Mast 3 (Autodesk Fusion 360 design; units mm, degrees)
Autodesk Fusion 360 part; units mm, degrees
sketch "Sketch1" plane through (0, 0, 0) normal (0, 0, 1) x (1, 0, 0)
  circle A0 centre (0, 0) radius 33
  circle A1 centre (0, 0) radius 32
  circle A2 centre (0, 0) radius 30
  circle A3 centre (0, 0) radius 16.2
  dimension "d1" = 66
  dimension "d2" = -1
  dimension "d3" = -3
  dimension "d10" = 60
  dimension "d15" = 32.4
  constraint coincident A0.centre A1.centre
  measures "d1" diameter of A0
  measures "d10" diameter of A2
  measures "d15" diameter of A3
extrude "Extrude1" add sketch "Sketch1" along normal blind 17 contours A0 | A1 | A2
extrude "Extrude2" cut sketch "Sketch1" along normal blind 15 contours A2 | A3
extrude "Extrude3" cut sketch "Sketch1" along normal blind 2 contours A1
sketch "Sketch2" plane through (0, 0, 15) normal (0, 0, -1) x (1, 0, 0)
  circle A0 centre (0, 0) radius 30
  line L0 (0, 0) -> (-30, 0) construction
  line L1 (-30, 5) -> (-29.5804, 5)
  line L2 (-16, 2.6667) -> (-16, -2.6667)
  line L3 (-29.5804, -5) -> (-30, -5)
  line L4 (-30, -5) -> (-30, 5)
  circle A1 centre (0, 0) radius 16.2
  line L5 (-30, 5) -> (0, 0) construction
  line L6 (-30, -5) -> (0, 0) construction
  line L7 (-30, 5) -> (-16, 2.6667)
  line L8 (-30, -5) -> (-16, -2.6667)
  dimension "d11" = 10
  dimension "d16" = 14
  constraint coincident A0.centre L0.start
  constraint coincident A0 L0.end
  constraint horizontal L0
  constraint horizontal L1
  constraint vertical L2
  constraint horizontal L3
  constraint vertical L4
  constraint coincident L0.end L4
  constraint midpoint L0.end L4
  constraint coincident L5 L2.start
  constraint coincident L6 L2.end
  constraint coincident A0 L1.end
  constraint coincident A0 L3.start
  measures "d11" distance of L1.start L3.end
  measures "d16" distance of L0.end L2
extrude "Extrude4" add sketch "Sketch2" along normal blind 8 contours A0 L2 A1 L7 L8 | L2 A1 picked at (-20.7852, 0) picked at (-16.0592, 0.283)
sketch "Sketch3" plane through (-16, 0, 0) normal (1, 0, 0) x (0, 1, 0)
  line L0 (-2.5377, 15) -> (-2.6667, 15)
  line L1 (-2.6667, 15) -> (-2.6667, 7)
  line L2 (-2.6667, 7) -> (2.6667, 7)
  line L3 (2.6667, 7) -> (2.6667, 15)
  circle A0 centre (0, 10) radius 2.5
  line L4 (2.6667, 15) -> (2.5377, 15)
  line L5 (2.5377, 15) -> (-2.5377, 15)
  line L6 (0, 0) -> (0, 15) construction
  dimension "d17" = 5
  dimension "d19" = 10
  constraint coincident L6.start origin
  constraint midpoint L5 L6.end
  constraint coincident A0.centre L6
  measures "d17" diameter of A0
  measures "d19" distance of L6.start A0.centre
extrude "Extrude5" cut sketch "Sketch3" against normal through all contours A0
